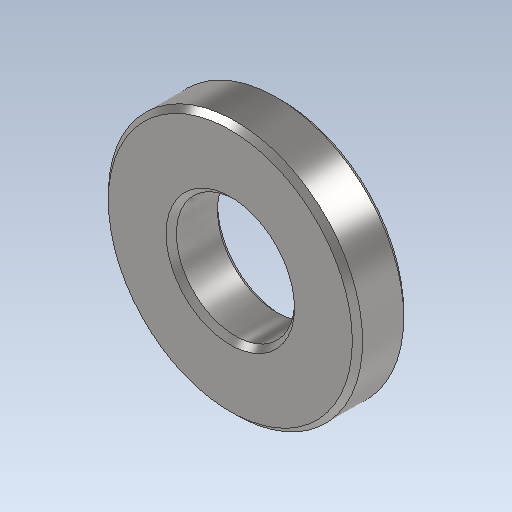
# Autodesk Inventor part: Кольцо поршень-шток низ_CPY
Saved by Autodesk Inventor 2021 (Build 250183000, 183)
## iProperties
Created: 2020-11-21
Part Number: Кольцо поршень-шток низ_CPY
Material: Сталь, мягкая
Document SubType Name: Modeling
Designer: Тимоха
Mass: 987.447 g
Surface Area: 205.208 cm^2
Volume: 125.789 cm^3
Density: 7.85 g/cm^3
Appearance: С умеренной полировкой
Author: Тимоха
Autodesk Inventor part; units mm, degrees
ref_plane "YZ Plane" through (0, 0, 0) normal (1, 0, 0) x (0, 1, 0)
ref_plane "XZ Plane" through (0, 0, 0) normal (0, 1, 0) x (-1, 0, 0)
ref_plane "XY Plane" through (0, 0, 0) normal (0, 0, 1) x (1, 0, 0)
sketch "Эскиз1" plane through (0, 0, 0) normal (0, 0, 1) x (1, 0, 0)
  circle A0 centre (0, 0) radius 49.5
  circle A1 centre (0, 0) radius 23
  dimension "d0" = 99
  dimension "d1" = 46
  constraints: 2 centre point, 2 coincident
  measures "d0" diameter of A0
  measures "d1" diameter of A1
extrude "Выдавливание1" add sketch "Эскиз1" along normal blind 20
chamfer "Фаска1" distance 2 angle 45 4 edges at (-23, 0, 20) (-49.5, 0, 20) (-23, 0, 0) (-49.5, 0, 0)
